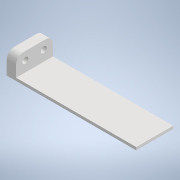
# Autodesk Inventor part: arms-3dp
Saved by Autodesk Inventor 2021 (Build 250183000, 183)
## iProperties
Created: 2021-03-27
Part Number: arms-3dp
Material: Generic
Document SubType Name: Modeling
Designer: ASUS
Density: 1 g/cm^3
Appearance: Default
Author: ASUS
Autodesk Inventor part; units mm, degrees
ref_plane "YZ Plane" through (0, 0, 0) normal (1, 0, 0) x (0, 1, 0)
ref_plane "XZ Plane" through (0, 0, 0) normal (0, 1, 0) x (-1, 0, 0)
ref_plane "XY Plane" through (0, 0, 0) normal (0, 0, 1) x (1, 0, 0)
sketch "Sketch1" plane through (0, 0, 0) normal (0, 1, 0) x (-1, 0, 0)
  line L0 (0, 0) -> (70, 0)
  line L1 (70, 0) -> (70, -20)
  line L2 (70, -20) -> (0, -20)
  line L3 (0, -20) -> (0, 0)
  dimension "d0" = 20
  dimension "d1" = 70
  constraints: 8 end point, 2 parallel, 1 horizontal, 1 perpendicular
  measures "d0" distance of L2.end L0.start
  measures "d1" distance of L1.end L2.end
extrude "Extrusion1" add sketch "Sketch1" along normal blind 1.5
sketch "Sketch2" plane through (0, 1.5, 0) normal (0, 1, 0) x (1, 0, 0)
  line L0 (-70, 0) -> (0, 0) projected
  line L1 (0, 20) -> (-70, 20) projected
  line L2 (-70, 0) -> (-65, 0)
  line L3 (-65, 0) -> (-65, 20)
  line L4 (-65, 20) -> (-70, 20)
  line L5 (-70, 20) -> (-70, 0)
  dimension "d4" = 5
  constraints: 8 end point, 2 parallel, 1 horizontal, 1 perpendicular, 1 point on line
  measures "d4" distance between parallel lines of L5 L3
extrude "Extrusion2" add sketch "Sketch2" along normal blind 10
sketch "Sketch3" plane through (-65, 1.5, 0) normal (1, 0, 0) x (0, 0, -1)
  circle A0 centre (5, 5.6701) radius 1.6
  circle A1 centre (15, 5.6701) radius 1.6
  point P0 (0, -1.5)
  dimension "d7" = 10
  dimension "d8" = 5
  dimension "d9" = 3.2
  constraints: 2 centre point, 1 equal radius
  measures "d7" distance of A0.centre A1.centre
  measures "d8" horizontal distance of point (0, -1.5) A0.centre
  measures "d9" diameter of A1
extrude "Extrusion3" cut sketch "Sketch3" against normal up to surface (5 mm away)
fillet "Fillet1" radius 4 2 edges at (-67.5, 11.5, -20) (-67.5, 11.5, 0)
ref_plane "Work Plane1" through (-70, 0, -10) normal (0, 0, 1) x (1, 0, 0)
sketch "Sketch4" plane through (-70, 0, -10) normal (0, 0, 1) x (1, 0, 0)
  line L0 (70, 0) -> (0, 0) projected
  line L1 (64, 0) -> (68, 0)
  line L2 (68, 0) -> (68, -4)
  line L3 (68, -4) -> (64, -4)
  line L4 (64, -4) -> (64, 0)
  circle A0 centre (66, -2) radius 1
  line L5 (70, 0) -> (70, 1.5) projected
  dimension "d13" = 2
  dimension "d14" = 4
  dimension "d15" = 2
  dimension "d16" = 2
  dimension "d17" = 2
  dimension "d18" = 2
  constraints: 8 end point, 2 parallel, 1 centre point, 1 horizontal, 1 perpendicular, 1 point on line
  measures "d13" diameter of A0
  measures "d14" distance of L2.end L3.end
  measures "d15" distance from line of L0 A0.centre
  measures "d16" distance from line of L3 A0.centre
  measures "d17" horizontal distance of L3.end A0.centre
  measures "d18" distance between parallel lines of L5 L2
extrude "Extrusion4" add sketch "Sketch4" along normal mid plane 3
fillet "Fillet2" radius 2 2 edges at (-2, -4, -10) (-6, -4, -10)
fillet "Fillet3" radius 7 2 edges at (0, 0.75, 0) (0, 0.75, -20)
body "Solid1"
